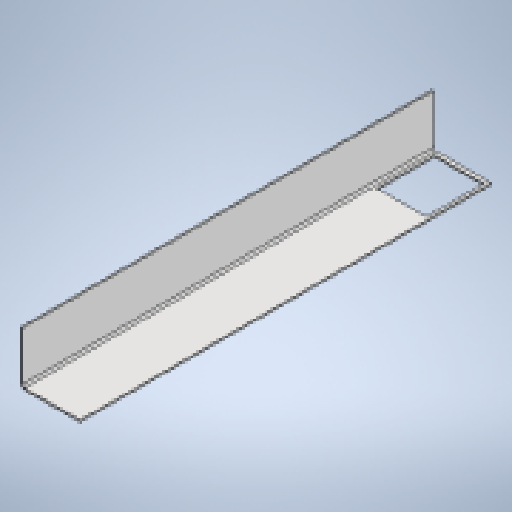
# Autodesk Inventor part: PNS 753 FDS 1200 FLANGE 3
Saved by Autodesk Inventor 2025.1 (Build 291241020, 241B)
## iProperties
Created: 2025-06-24
Part Number: PNS 753 FDS 1200 FLANGE 3
Material: Stainless Steel
Description: DIE16(5)|\ 90°|corrY -___°|X_____|bom___
Document SubType Name: Sheet Metal
Designer: user
Mass: 1762.25 g
Surface Area: 2283.33 cm^2
Volume: 220.281 cm^3
Density: 8 g/cm^3
Sheet Metal Rule: AISI304 2mm Die16
Sheet Metal Width: 0.000 mm
Sheet Metal Length: 0.000 mm
Sheet Metal Area: 0.000 mm^2
Appearance: Default
Author: user
Autodesk Inventor part; units mm, degrees
ref_plane "YZ Plane" through (0, 0, 0) normal (1, 0, 0) x (0, 1, 0)
ref_plane "XZ Plane" through (0, 0, 0) normal (0, 1, 0) x (-1, 0, 0)
ref_plane "XY Plane" through (0, 0, 0) normal (0, 0, 1) x (1, 0, 0)
sketch "Sketch1" plane through (0, 0, 0) normal (0, 0, 1) x (1, 0, 0)
  line L0 (-36, -250) -> (36, -250)
  line L1 (36, -250) -> (36, 250)
  line L2 (36, 250) -> (-36, 250)
  line L3 (-36, 250) -> (-36, -250)
  line L4 (-36, -250) -> (36, 250) construction
  line L5 (36, -250) -> (-36, 250) construction
  point P0 (0, 0)
  dimension "d154" = 72
  dimension "d155" = 500
  measures "d154" distance of L1.end L2.end
  measures "d155" distance of L0.end L1.end
extrude "Plate5" add sketch "Sketch1" along normal blind 2
sketch "Sketch7" plane through (-34, -250, 0) normal (-1, 0, 0) x (0, -1, 0)
  line L0 (-500, 0) -> (0, 0)
  line L1 (0, 0) -> (0, 64)
  line L2 (0, 64) -> (-500, 64)
  line L3 (-500, 64) -> (-500, 0)
  constraints: 6 end point, 1 horizontal, 1 perpendicular, 1 vertical
edge flange "Flange3" height 64 angle 90 thickness 2 bend radius 2.75 thickness toward (-1, 0, 0) relief round relief width 2 relief depth 1 edges at (-36, 0, 2) wall of the first edge with corners at (-34, 250, 0) (-34, -250, 0) (-34, -250, 64) (-34, 250, 64)
bend "Bend3"
corner "Corner3"
body "Solid3"
